Autodesk Inventor part; units mm, degrees
(part 2 of 2)
  spline S160 degree 2 poles (-14.5711, -12.6665) (-14.9899, -12.6665) (-15.46, -13.0313) (-15.46, -13.3549) knots 0 0 0 1 2 2 2
  spline S161 degree 2 poles (-15.46, -13.3549) (-15.46, -13.5502) (-15.2981, -13.9047) (-15.1723, -14.0408) knots 0 0 0 1 2 2 2
  line L273 (-15.1723, -14.0408) -> (-15.1723, -14.064)
  line L274 (-15.1723, -14.064) -> (-15.6218, -14.064)
  spline S162 degree 2 poles (-15.6218, -14.064) (-15.6501, -14.0049) (-15.7297, -13.8251) (-15.7477, -13.7531) knots 0 0 0 1 2 2 2
  spline S163 degree 2 poles (-15.7477, -13.7531) (-15.7785, -13.6504) (-15.8093, -13.4885) (-15.8093, -13.3627) knots 0 0 0 1 2 2 2
  spline S164 degree 2 poles (-14.566, -16.3837) (-15.1671, -16.3837) (-15.8222, -15.8057) (-15.8222, -15.3227) knots 0 0 0 1 2 2 2
  spline S165 degree 2 poles (-15.8222, -15.3227) (-15.8222, -14.8269) (-15.1466, -14.2592) (-14.566, -14.2592) knots 0 0 0 1 2 2 2
  spline S166 degree 2 poles (-14.566, -14.2592) (-13.97, -14.2592) (-13.3098, -14.8449) (-13.3098, -15.3227) knots 0 0 0 1 2 2 2
  spline S167 degree 2 poles (-13.3098, -15.3227) (-13.3098, -15.8057) (-13.9675, -16.3837) (-14.566, -16.3837) knots 0 0 0 1 2 2 2
  spline S168 degree 2 poles (-14.566, -15.9701) (-14.1036, -15.9701) (-13.6541, -15.6335) (-13.6541, -15.3227) knots 0 0 0 1 2 2 2
  spline S169 degree 2 poles (-13.6541, -15.3227) (-13.6541, -15.0119) (-14.1036, -14.6728) (-14.566, -14.6728) knots 0 0 0 1 2 2 2
  spline S170 degree 2 poles (-14.566, -14.6728) (-15.0156, -14.6728) (-15.478, -15.0119) (-15.478, -15.3227) knots 0 0 0 1 2 2 2
  spline S171 degree 2 poles (-15.478, -15.3227) (-15.478, -15.631) (-15.0233, -15.9701) (-14.566, -15.9701) knots 0 0 0 1 2 2 2
  line L275 (-15.7554, -19.492) -> (-14.3785, -19.492)
  spline S172 degree 2 poles (-14.3785, -19.492) (-14.2141, -19.492) (-13.9341, -19.4663) (-13.857, -19.4252) knots 0 0 0 1 2 2 2
  spline S173 degree 2 poles (-13.857, -19.4252) (-13.7722, -19.3841) (-13.69, -19.2274) (-13.69, -19.0913) knots 0 0 0 1 2 2 2
  spline S174 degree 2 poles (-13.69, -19.0913) (-13.69, -18.968) (-13.8416, -18.6854) (-13.9854, -18.5364) knots 0 0 0 1 2 2 2
  spline S175 degree 2 poles (-13.9854, -18.5364) (-14.0214, -18.539) (-14.1216, -18.5441) (-14.1884, -18.5441) knots 0 0 0 1 2 2 2
  line L276 (-14.1884, -18.5441) -> (-15.7554, -18.5441)
  line L277 (-15.7554, -18.5441) -> (-15.7554, -18.1433)
  line L278 (-15.7554, -18.1433) -> (-14.3785, -18.1433)
  spline S176 degree 2 poles (-14.3785, -18.1433) (-14.2141, -18.1433) (-13.9341, -18.1177) (-13.857, -18.0766) knots 0 0 0 1 2 2 2
  spline S177 degree 2 poles (-13.857, -18.0766) (-13.7722, -18.0354) (-13.69, -17.8787) (-13.69, -17.7426) knots 0 0 0 1 2 2 2
  spline S178 degree 2 poles (-13.69, -17.7426) (-13.69, -17.6142) (-13.8519, -17.329) (-13.9777, -17.1954) knots 0 0 0 1 2 2 2
  line L279 (-13.9777, -17.1954) -> (-15.7554, -17.1954)
  line L280 (-15.7554, -17.1954) -> (-15.7554, -16.7947)
  line L281 (-15.7554, -16.7947) -> (-13.3766, -16.7947)
  line L282 (-13.3766, -16.7947) -> (-13.3766, -17.1954)
  line L283 (-13.3766, -17.1954) -> (-13.6386, -17.1954)
  spline S179 degree 2 poles (-13.6386, -17.1954) (-13.4819, -17.3521) (-13.3098, -17.6604) (-13.3098, -17.8454) knots 0 0 0 1 2 2 2
  spline S180 degree 2 poles (-13.3098, -17.8454) (-13.3098, -18.056) (-13.5025, -18.3822) (-13.7208, -18.467) knots 0 0 0 1 2 2 2
  spline S181 degree 2 poles (-13.7208, -18.467) (-13.5179, -18.6494) (-13.3098, -18.9936) (-13.3098, -19.194) knots 0 0 0 1 2 2 2
  spline S182 degree 2 poles (-13.3098, -19.194) (-13.3098, -19.3481) (-13.4049, -19.5999) (-13.5128, -19.6924) knots 0 0 0 1 2 2 2
  spline S183 degree 2 poles (-13.5128, -19.6924) (-13.6207, -19.7874) (-13.9443, -19.8928) (-14.1884, -19.8928) knots 0 0 0 1 2 2 2
  line L284 (-14.1884, -19.8928) -> (-15.7554, -19.8928)
  line L285 (-15.7554, -19.8928) -> (-15.7554, -19.492)
  point P0 (0, 0)
  constraints: 2 other
extrude "Extrusion8" add sketch "Sketch9" along normal blind 0.5
sketch "Sketch10" plane through (0, 2, 0) normal (0, 1, 0) x (1, 0, 0)
  line L0 (29.0932, 58.6501) -> (-22.9068, 58.6501) projected
  line L1 (-22.9068, 58.6501) -> (-17.9068, 58.6501)
  line L2 (-22.9068, 58.6501) -> (-22.9068, 53.6501)
  line L3 (-22.9068, 58.6501) -> (-22.9068, -60.3499) projected
  line L4 (-22.9068, 53.6501) -> (-17.9068, 58.6501)
  line L5 (-17.9068, 58.6501) -> (-15.9068, 58.6501)
  line L6 (-15.9068, 58.6501) -> (-22.9068, 51.6501)
  line L7 (-22.9068, 51.6501) -> (-22.9068, 46.6501)
  line L8 (-22.9068, 46.6501) -> (-10.9068, 58.6501)
  line L9 (-10.9068, 58.6501) -> (-8.9068, 58.6501)
  line L10 (-8.9068, 58.6501) -> (-22.9068, 44.6501)
  line L11 (-22.9068, 44.6501) -> (-22.9068, 39.6501)
  line L12 (-22.9068, 39.6501) -> (-3.9068, 58.6501)
  line L13 (-3.9068, 58.6501) -> (-1.9068, 58.6501)
  line L14 (-1.9068, 58.6501) -> (-22.9068, 37.6501)
  point P0 (0, 0)
  dimension "d36" = 5
  dimension "d37" = 5
  dimension "d38" = 2
  dimension "d39" = 5
  dimension "d40" = 2
  dimension "d41" = 5
  dimension "d42" = 2
  constraints: 26 end point, 12 point on line, 2 parallel
  measures "d36" distance of L0.end L1.end
  measures "d37" distance of L0.end L2.end
  measures "d38" distance of L1.end L5.end
  measures "d39" distance of L6.end L7.end
  measures "d40" distance of L8.end L9.end
  measures "d41" distance of L10.end L11.end
  measures "d42" distance of L12.end L13.end
extrude "Extrusion9" cut sketch "Sketch10" against normal blind 0.5 contours L14 L3 L12 L0 | L10 L3 L8 L0 | L6 L3 L4 L0
chamfer "Chamfer3" distance 1 angle 45 8 edges at (27.0932, 2, -1.1501) (26.0932, 2, -22.6501) (14.0932, 2, -23.6501) (2.0932, 2, -22.6501) (1.0932, 2, -1.1501) (2.0932, 2, 20.3499) (14.0932, 2, 21.3499) (26.0932, 2, 20.3499)
equation "\"BendRadius\" = Thickness"
equation "\"BendReliefWidth\" = Thickness"
equation "\"BendReliefDepth\" = 0.5 * Thickness"
equation "\"CornerReliefSize\" = 4 * Thickness"
equation "\"MinimumRemnant\" = 2 * Thickness"
equation "\"TransitionRadius\" = BendRadius"
equation "\"JacobiRadiusSize\" = BendRadius"
equation "\"GapSize\" = Thickness"
equation "\"Thickness\" = 0.5"
body "Solid1"
